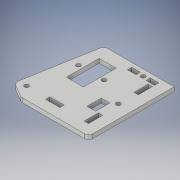
# Autodesk Inventor part: 板子1
Saved by Autodesk Inventor 2017 (Build 210142000, 142)
## iProperties
Part Number: 板子1
Material: 一般
Document SubType Name: Modeling
Designer: User
Density: 1 g/cm^3
Appearance: 預設
Author: User
Autodesk Inventor part; units mm, degrees
ref_plane "YZ Plane" through (0, 0, 0) normal (1, 0, 0) x (0, 1, 0)
ref_plane "XZ Plane" through (0, 0, 0) normal (0, 1, 0) x (-1, 0, 0)
ref_plane "XY Plane" through (0, 0, 0) normal (0, 0, 1) x (1, 0, 0)
sketch "草圖1" plane through (0, 0, 0) normal (0, 1, 0) x (-1, 0, 0)
  line L0 (24.1962, 30) -> (-19.5, 30)
  line L1 (-22.5, 27) -> (-22.5, -27)
  line L2 (-22.5, -30) -> (24.1827, -30)
  line L3 (25, 30) -> (17.3, 30)
  line L4 (25.6962, 29.5981) -> (33.7194, 24.9658)
  line L5 (-19.5, -30) -> (26.7, -30)
  line L6 (27.1371, -27.5209) -> (35.6587, 20.8071)
  line L7 (-14.8, -27) -> (-8.8, -27)
  line L8 (-8.8, -27) -> (-8.8, -24)
  line L9 (-8.8, -24) -> (-14.8, -24)
  line L10 (-14.8, -24) -> (-14.8, -27)
  line L11 (-14.8, -22.5) -> (-11.8, -22.5)
  line L12 (-11.8, -22.5) -> (-11.8, -12.5)
  line L13 (-11.8, -12.5) -> (-14.8, -12.5)
  line L14 (-14.8, -12.5) -> (-14.8, -22.5)
  line L15 (-11.8, -12.5) -> (-13.3, -12.5)
  circle A0 centre (-13.3, 0) radius 1.5
  line L16 (-11.8, 22.5) -> (-14.8, 22.5)
  line L17 (-14.8, 22.5) -> (-14.8, 12.5)
  line L18 (-14.8, 12.5) -> (-11.8, 12.5)
  line L19 (-11.8, 12.5) -> (-11.8, 22.5)
  circle A1 centre (-5.3, -25.5) radius 1.5
  line L20 (4.2, -24) -> (-1.8, -24)
  line L21 (-1.8, -24) -> (-1.8, -27)
  line L22 (-1.8, -27) -> (4.2, -27)
  line L23 (4.2, -27) -> (4.2, -24)
  line L24 (9.2, -21) -> (21.2, -21)
  line L25 (21.2, -21) -> (21.2, 2)
  line L26 (21.2, 2) -> (9.2, 2)
  line L27 (9.2, 2) -> (9.2, -21)
  line L28 (9.2, -21) -> (9.2, -9.5)
  circle A2 centre (6.2, -9.5) radius 1.5
  circle A3 centre (24.2, -9.5) radius 1.5
  line L29 (5, 19.8) -> (15, 19.8)
  line L30 (15, 19.8) -> (15, 22.8)
  line L31 (15, 22.8) -> (5, 22.8)
  line L32 (5, 22.8) -> (5, 19.8)
  line L33 (-22.5, -30) -> (-22.5, -27)
  line L34 (-22.5, -27) -> (-14.8, -27)
  line L35 (-3.8, 12.5) -> (-9.8, 12.5)
  line L36 (-9.8, 12.5) -> (-9.8, 2.5)
  line L37 (-9.8, 2.5) -> (-3.8, 2.5)
  line L38 (-3.8, 2.5) -> (-3.8, 12.5)
  line L39 (15, 22.8) -> (15, 21.3)
  line L40 (15, 21.3) -> (29.9, 21.3)
  circle A4 centre (29.9, 21.3) radius 1.5
  arc A5 (25.6962, 29.5981) -> (24.1962, 30) centre (24.1962, 27) ccw
  arc A6 (35.6587, 20.8071) -> (33.7194, 24.9658) centre (31.7194, 21.5017) ccw
  arc A7 (24.1827, -30) -> (27.1371, -27.5209) centre (24.1827, -27) ccw
  arc A8 (-22.5, -27) -> (-19.5, -30) centre (-19.5, -27) ccw
  arc A9 (-19.5, 30) -> (-22.5, 27) centre (-19.5, 27) ccw
  point P0 (-22.5, 30)
  point P1 (25, -30)
  dimension "d0" = 60
  dimension "d1" = 47.5
  dimension "d43" = 49.2
  dimension "d44" = 110
  dimension "d46" = 3
  dimension "d47" = 1.5
  dimension "d48" = 3
  dimension "d49" = 10
  dimension "d50" = 3
  dimension "d51" = 1.5
  dimension "d53" = 3
  dimension "d54" = 3
  dimension "d55" = 10
  dimension "d56" = 3
  dimension "d61" = 3
  dimension "d62" = 6
  dimension "d63" = 3
  dimension "d67" = 12
  dimension "d68" = 23
  dimension "d69" = 11.5
  dimension "d72" = 3
  dimension "d73" = 3
  dimension "d74" = 10
  dimension "d75" = 3
  dimension "d76" = 3
  dimension "d77" = 7.7
  dimension "d78" = 6
  dimension "d79" = 10
  dimension "d80" = 32.5
  dimension "d81" = 12.7
  dimension "d82" = 14.9
  dimension "d83" = 3
  dimension "d84" = 3
  dimension "d85" = 4
  constraints: 82 end point, 12 perpendicular, 10 centre point, 10 point on circle, 10 point on line, 10 tangent, 9 parallel, 3 equal radius, 3 horizontal, 3 midpoint, 1 coincident
  measures "d0" distance of point (25, -30) L3.start
  measures "d1" distance of L3.start point (-22.5, 30)
  measures "d43" distance of L2.start L5.end
  measures "d44" angle of L6 L4
  measures "d46" distance of L9.end L10.end
  measures "d47" distance of L9.end L11.start
  measures "d48" distance of L11.start L11.end
  measures "d49" distance of L11.end L15.start
  measures "d50" distance of L15.start L14.start
  measures "d51" distance of L15.start L15.end
  measures "d53" diameter of A0
  measures "d54" distance of L18.start L18.end
  measures "d55" distance of L18.end L19.end
  measures "d56" distance of L19.end L17.start
  measures "d61" diameter of A1
  measures "d62" distance of L23.end L20.end
  measures "d63" distance of L20.end L22.start
  measures "d67" distance of L27.end L25.start
  measures "d68" distance of L25.start L25.end
  measures "d69" distance of L27.end L28.end
  measures "d72" diameter of A2
  measures "d73" diameter of A3
  measures "d74" distance of L32.end L29.end
  measures "d75" distance of L32.start L32.end
  measures "d76" distance of L2.start L33.end
  measures "d77" distance of L33.end L34.end
  measures "d78" distance of L36.end L37.end
  measures "d79" distance of L37.end L35.start
  measures "d80" distance between parallel lines of L2 L37
  measures "d81" distance between parallel lines of L1 L36
  measures "d82" distance of L39.end L40.end
  measures "d83" diameter of A4
  measures "d84" radius of A5
  measures "d85" radius of A6
extrude "擠出2" add sketch "草圖1" along normal mid plane 3
